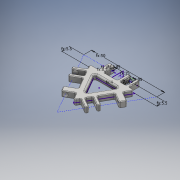
# Autodesk Inventor part: triangle
Saved by Autodesk Inventor 2016 (Build 200138000, 138)
## iProperties
Created: 2016-11-12
Part Number: triangle
Material: Generic
Document SubType Name: Modeling
Designer: Chris
Density: 1 g/cm^3
Appearance: Default
Author: Chris
Autodesk Inventor part; units mm, degrees
ref_plane "XZ Plane" through (0, 0, 0) normal (0, 1, 0) x (-1, 0, 0)
ref_plane "XY Plane" through (0, 0, 0) normal (0, 0, 1) x (1, 0, 0)
sketch "Sketch1" plane through (0, 0, 0) normal (0, 0, 1) x (1, 0, 0)
  line L0 (25, 14.4338) -> (0, -28.8675) construction
  line L1 (0, -28.8675) -> (-25, 14.4338) construction
  line L2 (-25, 14.4338) -> (25, 14.4338) construction
  line L3 (15.4737, 8.9338) -> (0, -17.8675)
  line L4 (0, -17.8675) -> (-15.4737, 8.9338)
  line L5 (-15.4737, 8.9338) -> (15.4737, 8.9338)
  line L6 (-7.5, 14.4338) -> (7.5, 14.4338) construction
  line L7 (5.475, 14.4338) -> (9.525, 14.4338) construction
  line L8 (-9.475, 14.4338) -> (-5.525, 14.4338) construction
  line L9 (8.5455, 4.9338) -> (0, -9.8675)
  line L10 (0, -9.8675) -> (-8.5455, 4.9338)
  line L11 (-8.5455, 4.9338) -> (8.5455, 4.9338)
  point P0 (0, 0)
  point P1 (0, 0)
  point P2 (0, 14.4338)
  dimension "d0" = 50
  dimension "d2" = 15
  dimension "d4" = 4.05
  dimension "d5" = 5.5
  dimension "d6" = 3.95
  dimension "d7" = 4
  dimension "d18" = 5.5
  constraints: 24 end point, 7 coincident, 4 horizontal, 4 midpoint, 1 collinear, 11 other
  measures "d0" distance of L1.end L0.start
  measures "d2" distance of L6.start L6.end
  measures "d4" distance of L7.start L7.end
  measures "d5" distance between parallel lines of L5 L7
  measures "d6" distance of L8.start L8.end
  measures "d7" distance between parallel lines of L5 L11
  measures "d18" distance between parallel lines of L5 L2
extrude "Extrusion1" add sketch "Sketch1" along normal mid plane 4
sketch "Sketch2" plane through (0, 0, 0) normal (1, 0, 0) x (0, 1, 0)
  line L0 (8.9338, 2) -> (8.9338, -2) construction
  line L1 (8.9338, -2) -> (8.9338, 2) construction
  line L2 (8.9338, 2) -> (13.9338, 2) construction
  line L3 (12.9338, -2) -> (8.9338, -2) construction
  line L4 (8.9338, -2) -> (8.9338, 2) construction
  arc A0 (14.4338, -2) -> (14.4338, 2) centre (14.4338, 0) ccw
  line L5 (14.4338, -2) -> (8.9338, -2)
  line L6 (8.9338, -2) -> (8.9338, 2)
  line L7 (8.9338, 2) -> (14.4338, 2)
  line L8 (14.4338, -2) -> (16.4338, -2)
  line L9 (16.4338, -2) -> (16.4338, 2)
  line L10 (16.4338, 2) -> (14.4338, 2)
  point P0 (0, 0)
  point P1 (14.4338, 0)
  point P2 (14.4338, 0)
  constraints: 18 end point, 5 perpendicular, 3 horizontal, 3 tangent, 2 coincident, 2 point on circle, 2 point on line, 1 centre point, 1 parallel
ref_plane "Work Plane1" through (-9.475, 14.4338, 0) normal (1, 0, 0) x (0, 1, 0)
ref_plane "Work Plane2" through (-5.525, 14.4338, 0) normal (1, 0, 0) x (0, 1, 0)
ref_plane "Work Plane3" through (5.475, 14.4338, 0) normal (1, 0, 0) x (0, 1, 0)
ref_plane "Work Plane4" through (9.525, 14.4338, 0) normal (1, 0, 0) x (0, 1, 0)
extrude "Extrusion2" add sketch "Sketch2" along normal up to surface (3.95 mm away) from surface at -9.475
ref_plane "Work Plane5" through (3.475, 14.4338, 0) normal (1, 0, 0) x (0, 1, 0)
ref_plane "Work Plane6" through (11.525, 14.4338, 0) normal (1, 0, 0) x (0, 1, 0)
extrude "Extrusion3" add sketch "Sketch2" along normal up to surface (2 mm away) from surface at 3.475
extrude "Extrusion4" add sketch "Sketch2" along normal up to surface (2 mm away) from surface at 9.525
sketch "Sketch3" plane through (0, 0, 0) normal (0, 0, 1) x (1, 0, 0)
  line L0 (-9.475, 15.9338) -> (-9.475, 14.4338)
  line L1 (-5.525, 15.9338) -> (-5.525, 14.4338)
  line L2 (5.475, 15.9338) -> (5.475, 14.4338)
  line L3 (9.525, 15.9338) -> (9.525, 14.4338)
  line L4 (5.475, 14.4338) -> (9.525, 14.4338) construction
  line L5 (-7.5, 14.4338) -> (7.5, 14.4338) construction
  arc A0 (5.975, 14.4338) -> (5.475, 15.9338) centre (3.475, 14.4338) ccw
  arc A1 (9.525, 15.9338) -> (9.025, 14.4338) centre (11.525, 14.4338) ccw
  arc A2 (-8.975, 14.4338) -> (-9.475, 15.9338) centre (-11.475, 14.4338) ccw
  arc A3 (-5.525, 15.9338) -> (-6.025, 14.4338) centre (-3.525, 14.4338) ccw
  line L6 (9.025, 14.4338) -> (9.525, 14.4338)
  line L7 (5.975, 14.4338) -> (5.475, 14.4338)
  line L8 (-5.525, 14.4338) -> (-6.025, 14.4338)
  line L9 (-8.975, 14.4338) -> (-9.475, 14.4338)
  point P0 (0, 0)
  point P1 (5.475, 16.4338)
  dimension "d31" = 0.5
  dimension "d32" = 3
  dimension "d33" = 0.5
  constraints: 16 end point, 8 point on circle, 5 collinear, 5 point on line, 4 centre point, 4 coincident, 4 vertical, 3 equal radius, 2 horizontal alignment
  measures "d31" distance of L2.end L7.start
  measures "d32" diameter of point (-9.475, 15.934) L9
  measures "d33" distance of L9.start L0.end
revolve "Revolution1" cut sketch "Sketch3" angle 360 about axis through (-8.975, 14.4338, 0) along (-1, 0, 0) contours A2 L9 L0 | L1 L8 A3
revolve "Revolution2" add sketch "Sketch3" angle 360 about axis through (5.975, 14.4338, 0) along (-1, 0, 0) contours A0 L7 L2 | L3 L6 A1
pattern_circular "Circular Pattern1" count 3 over 360 about axis through (0, 0, -10) along (0, 0, 1) of "Extrusion4", "Extrusion3", "Extrusion2", "Revolution1", "Revolution2"
fillet "Fillet2" radius 1 6 edges at (15.4737, 8.9338, 0) (-15.4737, 8.9338, 0) (0, -17.8675, 0) (8.5455, 4.9338, 0) (-8.5455, 4.9338, 0) (0, -9.8675, 0)
fillet "Fillet3" radius 0.75 36 edges at (2.9744, -12.7158, 0) (4.9994, -9.2084, 0) (5.9994, -7.4763, 0) (10.4994, 0.3179, 0) (12.4744, 3.7387, 0) (9.525, 8.9338, 0) (5.475, 8.9338, 0) (3.475, 8.9338, 0) (-5.525, 8.9338, 0) (-9.475, 8.9338, 0) (-12.4994, 3.782, 0) (-10.4744, 0.2746, 0) (-9.4744, -1.4574, 0) (-4.9744, -9.2517, 0) (-2.9994, -12.6725, 0) (-13.4994, 5.5141, 0) (11.525, 8.9338, 0) (1.9744, -14.4478, 0) (8.4696, -18.1978, 0) (9.4696, -16.4658, 0) (11.4946, -12.9584, 0) (12.4946, -11.2263, 0) (16.9946, -3.4321, 0) (18.9696, -0.0113, 0) (11.525, 16.4338, 0) (9.525, 16.4338, 0) (5.475, 16.4338, 0) (3.475, 16.4338, 0) (-5.525, 16.4338, 0) (-9.475, 16.4338, 0) (-19.9946, 1.7641, 0) (-18.9946, 0.032, 0) (-16.9696, -3.4754, 0) (-15.9696, -5.2074, 0) (-11.4696, -13.0017, 0) (-9.4946, -16.4225, 0)
fillet "Fillet4" radius 1 12 edges at (4.2728, -2.4669, -2) (0, -8.8675, -2) (-4.2728, -2.4669, -2) (-7.6795, 4.4338, -2) (0, 4.9338, -2) (7.6795, 4.4338, -2) (0, 4.9338, 2) (-7.6795, 4.4338, 2) (-4.2728, -2.4669, 2) (0, -8.8675, 2) (4.2728, -2.4669, 2) (7.6795, 4.4338, 2)
chamfer "Chamfer1" distance 0.4 angle 45 132 edges at (13.7285, 5.911, 2) (14.6077, 8.4338, 2) (13.0083, 8.9338, 2) (11.7447, 9.1534, 2) (11.525, 12.6838, 2) (11.3053, 16.2141, 2) (9.525, 12.6838, 2) (9.3053, 9.1534, 2) (7.5, 8.9338, 2) (5.6947, 9.1534, 2) (5.475, 12.6838, 2) (5.2553, 16.2141, 2) (3.475, 12.6838, 2) (3.2553, 9.1534, 2) (-1.025, 8.9338, 2) (-5.3053, 9.1534, 2) (-5.525, 12.6838, 2) (-5.7447, 16.2141, 2) (-7.5, 16.4338, 2) (-9.2553, 16.2141, 2) (-9.475, 12.6838, 2) (-9.6947, 9.1534, 2) (-11.9833, 8.9338, 2) (-14.6077, 8.4338, 2) (-14.241, 6.7987, 2) (-13.7994, 5.5945, 2) (-16.747, 3.6391, 2) (-19.6945, 1.6837, 2) (-15.747, 1.907, 2) (-12.5798, 3.4819, 2) (-11.4869, 2.0283, 2) (-10.7744, 0.355, 2) (-13.722, -1.6004, 2) (-16.6695, -3.5558, 2) (-12.722, -3.3324, 2) (-9.5548, -1.7575, 2) (-7.2244, -5.3546, 2) (-5.2744, -9.1713, 2) (-8.222, -11.1267, 2) (-11.1695, -13.0821, 2) (-10.4821, -14.7121, 2) (-9.4141, -16.1224, 2) (-6.247, -14.5475, 2) (-3.0798, -12.9725, 2) (-1.7452, -14.8448, 2) (0, -16.8675, 2) (1.2327, -15.7324, 2) (2.0548, -14.7479, 2) (5.222, -16.3228, 2) (8.3891, -17.8977, 2) (6.222, -14.5908, 2) (3.2744, -12.6354, 2) (3.9869, -10.9621, 2) (5.0798, -9.5084, 2) (8.247, -11.0834, 2) (11.4141, -12.6583, 2) (9.247, -9.3513, 2) (6.2994, -7.3959, 2) (8.2494, -3.5792, 2) (10.5798, 0.0178, 2) (13.747, -1.5571, 2) (16.9141, -3.132, 2) (17.9821, -1.7217, 2) (18.6695, -0.0917, 2) (15.722, 1.8637, 2) (12.7744, 3.8191, 2) (13.747, -1.5571, -2) (10.5798, 0.0178, -2) (8.2494, -3.5792, -2) (6.2994, -7.3959, -2) (9.247, -9.3513, -2) (11.4141, -12.6583, -2) (8.247, -11.0834, -2) (5.0798, -9.5084, -2) (3.9869, -10.9621, -2) (3.2744, -12.6354, -2) (6.222, -14.5908, -2) (8.3891, -17.8977, -2) (5.222, -16.3228, -2) (2.0548, -14.7479, -2) (1.2327, -15.7324, -2) (0, -16.8675, -2) (-1.7452, -14.8448, -2) (-3.0798, -12.9725, -2) (-6.247, -14.5475, -2) (-9.4141, -16.1224, -2) (-10.4821, -14.7121, -2) (-11.1695, -13.0821, -2) (-8.222, -11.1267, -2) (-5.2744, -9.1713, -2) (-7.2244, -5.3546, -2) (-9.5548, -1.7575, -2) (-12.722, -3.3324, -2) (-16.6695, -3.5558, -2) (-13.722, -1.6004, -2) (-10.7744, 0.355, -2) (-11.4869, 2.0283, -2) (-12.5798, 3.4819, -2) (-15.747, 1.907, -2) (-19.6945, 1.6837, -2) (-16.747, 3.6391, -2) (-13.7994, 5.5945, -2) (-14.241, 6.7987, -2) (-14.6077, 8.4338, -2) (-11.9833, 8.9338, -2) (-9.6947, 9.1534, -2) (-9.475, 12.6838, -2) (-9.2553, 16.2141, -2) (-7.5, 16.4338, -2) (-5.7447, 16.2141, -2) (-5.525, 12.6838, -2) (-5.3053, 9.1534, -2) (-1.025, 8.9338, -2) (3.2553, 9.1534, -2) (3.475, 12.6838, -2) (5.2553, 16.2141, -2) (5.475, 12.6838, -2) (5.6947, 9.1534, -2) (7.5, 8.9338, -2) (9.3053, 9.1534, -2) (9.525, 12.6838, -2) (11.3053, 16.2141, -2) (11.525, 12.6838, -2) (11.7447, 9.1534, -2) (13.0083, 8.9338, -2) (14.6077, 8.4338, -2) (13.7285, 5.911, -2) (12.7744, 3.8191, -2) (15.722, 1.8637, -2) (18.6695, -0.0917, -2) (17.9821, -1.7217, -2) (16.9141, -3.132, -2)
equation "\"d7\" = diam"
equation "\"d8\" = diam"
equation "\"d10\" = diam"
equation "\"d14\" = diam"
equation "\"d16\" = diam"
equation "\"diam\" = 4"
equation "\"dent\" = 0.5"
equation "\"matespace\" = 15"
equation "\"springwidth\" = 2"
equation "\"fingerwidth\" = 4"
equation "\"tolerance\" = 0.1"
equation "\"dentdiam\" = 3"
equation "\"springlength\" = 5.5"
body "Solid1"
